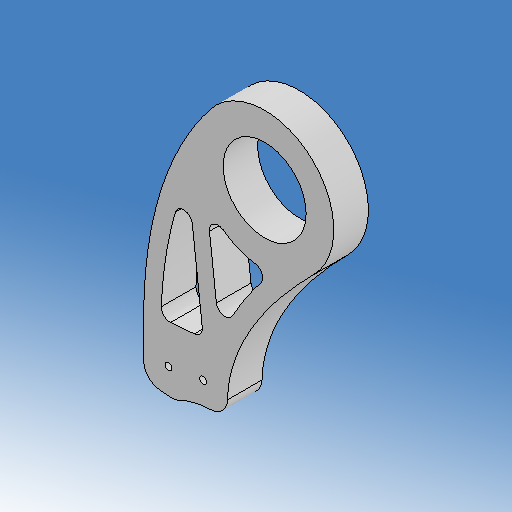
# Autodesk Inventor part: driveshaftsupport_A
Saved by Autodesk Inventor 2025 (Build 290162000, 162)
## iProperties
Created: 2023-03-01
Part Number: driveshaftsupport_A
Material: Generic
Document SubType Name: Modeling
Designer: ralph
Density: 1 g/cm^3
Appearance: Default
Author: ralph
Autodesk Inventor part; units mm, degrees
(part 1 of 2)
ref_plane "YZ Plane" through (0, 0, 0) normal (1, 0, 0) x (0, 1, 0)
ref_plane "XZ Plane" through (0, 0, 0) normal (0, 1, 0) x (-1, 0, 0)
ref_plane "Work Plane1" through (0, 0, 0) normal (0, 0, 1) x (1, 0, 0)
sketch "Sketch1" plane through (0, 0, 0) normal (0, 0, 1) x (1, 0, 0)
  arc A0 (-20.648, -102.4649) -> (-16.3515, -107.2084) centre (-14.4346, -101.1546) ccw
  arc A1 (-10.9828, -109.2489) -> (-16.3515, -107.2084) centre (-31.6865, -155.6385) ccw
  arc A2 (-10.9828, -109.2489) -> (-4.2979, -108.3017) centre (-8.3948, -103.4502) ccw
  arc A3 (0.8876, -104.599) -> (-4.2979, -108.3017) centre (21.0506, -138.319) ccw
  arc A4 (7.2668, -104.5186) -> (0.8876, -104.599) centre (4.1465, -110.049) ccw
  arc A5 (7.2668, -104.5186) -> (24.5776, -101.9869) centre (14.2875, -92.075) ccw
  arc A6 (30.7127, -100.2372) -> (24.5776, -101.9869) centre (29.151, -106.3922) ccw
  arc A7 (43.0033, -105.7359) -> (30.7127, -100.2372) centre (21.0506, -138.319) ccw
  arc A8 (43.0033, -105.7359) -> (57.752, -89.4091) centre (49.2125, -96.52) ccw
  arc A9 (57.752, -7.1109) -> (57.752, -89.4091) centre (107.1678, -48.26) ccw
  arc A10 (57.752, -7.1109) -> (57.752, 7.1109) centre (49.2125, 0) ccw
  arc A11 (57.752, 89.4091) -> (57.752, 7.1109) centre (107.1678, 48.26) ccw
  arc A12 (57.752, 89.4091) -> (46.7209, 107.3496) centre (49.2125, 96.52) ccw
  arc A13 (37.2777, 118.8104) -> (46.7209, 107.3496) centre (44.8601, 115.4372) ccw
  arc A14 (37.2777, 118.8104) -> (27.7131, 132.1679) centre (28.575, 122.682) ccw
  arc A15 (-1.8719, 154.7102) -> (27.7131, 132.1679) centre (25.2222, 159.584) ccw
  arc A16 (-1.8719, 154.7102) -> (-9.0898, 161.7077) centre (-11.1125, 152.4) ccw
  arc A17 (-57.3497, 188.5663) -> (-9.0898, 161.7077) centre (11.1567, 254.8735) ccw
  arc A18 (-57.3497, 188.5663) -> (-61.9125, 190.5) centre (-61.9125, 184.15) ccw
  line L0 (-61.9125, -74.837) -> (-61.9125, 190.5)
  arc A19 (-57.4675, -76.6522) -> (-61.9125, -74.837) centre (-61.9125, -81.187) ccw
  arc A20 (-57.4675, -76.6522) -> (-50.3955, -79.3664) centre (-50.8, -69.85) ccw
  arc A21 (-20.648, -102.4649) -> (-50.3955, -79.3664) centre (-49.1581, -108.4774) ccw
  line L1 (-54.9779, 170.3652) -> (-48.8256, 159.5987)
  arc A22 (-48.8539, 153.2488) -> (-48.8256, 159.5987) centre (-54.339, 156.4482) ccw
  arc A23 (-48.8539, 153.2488) -> (-49.1732, 139.4288) centre (-36.5125, 146.05) ccw
  arc A24 (-49.4382, 133.0844) -> (-49.1732, 139.4288) centre (-54.8001, 136.4861) ccw
  line L2 (-49.4382, 133.0844) -> (-55.0158, 124.2927)
  arc A25 (-57.9437, 125.1431) -> (-55.0158, 124.2927) centre (-56.3562, 125.1431) ccw
  line L3 (-57.9437, 125.1431) -> (-57.9437, 169.5776)
  arc A26 (-54.9779, 170.3652) -> (-57.9437, 169.5776) centre (-56.3562, 169.5776) ccw
  line L4 (-57.9437, 16.3803) -> (-57.9437, 88.2093)
  arc A27 (-48.4371, 93.7191) -> (-57.9437, 88.2093) centre (-51.5937, 88.2093) ccw
  line L5 (-48.4371, 93.7191) -> (25.1122, 51.5817)
  arc A28 (24.9048, 45.9631) -> (25.1122, 51.5817) centre (23.5339, 48.8268) ccw
  line L6 (24.9048, 45.9631) -> (-48.8518, 10.6528)
  arc A29 (-57.9437, 16.3803) -> (-48.8518, 10.6528) centre (-51.5937, 16.3803) ccw
  line L7 (-12.5571, -63.0775) -> (-11.8021, -62.3567)
  arc A30 (-6.8531, -63.0782) -> (-11.8021, -62.3567) centre (-9.6098, -64.6534) ccw
  line L8 (-6.8531, -63.0782) -> (0.9035, -76.6523)
  arc A31 (-1.2505, -78.8251) -> (0.9035, -76.6523) centre (-0.4748, -77.44) ccw
  line L9 (-1.2505, -78.8251) -> (-11.2752, -73.2112)
  arc A32 (-12.5571, -63.0775) -> (-11.2752, -73.2112) centre (-8.1726, -67.6708) ccw
  line L10 (8.063, -43.7132) -> (40.1759, -13.8303)
  arc A33 (42.6746, -15.7078) -> (40.1759, -13.8303) centre (41.2574, -14.9925) ccw
  arc A34 (42.6746, -15.7078) -> (35.0956, -43.2986) centre (107.1678, -48.26) ccw
  arc A35 (28.7606, -49.2125) -> (35.0956, -43.2986) centre (28.7606, -42.8625) ccw
  line L11 (28.7606, -49.2125) -> (10.2259, -49.2125)
  arc A36 (8.063, -43.7132) -> (10.2259, -49.2125) centre (10.2259, -46.0375) ccw
  arc A37 (0.0566, -90.8047) -> (0.0035, -91.7596) centre (14.2875, -92.075) ccw
  arc A38 (-5.1562, -94.1671) -> (0.0035, -91.7596) centre (-3.1707, -91.6895) ccw
  arc A39 (-5.1562, -94.1671) -> (-8.4369, -92.4585) centre (-11.1125, -101.6) ccw
  arc A40 (-12.4439, -88.97) -> (-8.4369, -92.4585) centre (-6.6532, -86.3642) ccw
  line L12 (-12.4439, -88.97) -> (-14.871, -83.5766)
  arc A41 (-12.6476, -81.54) -> (-14.871, -83.5766) centre (-13.4233, -82.9251) ccw
  line L13 (-12.6476, -81.54) -> (-1.5545, -87.7521)
  arc A42 (0.0566, -90.8047) -> (-1.5545, -87.7521) centre (-3.1058, -90.5224) ccw
  line L14 (35.1248, 3.9688) -> (-30.4467, 3.9688)
  arc A43 (-31.8177, 10.0075) -> (-30.4467, 3.9688) centre (-30.4467, 7.1438) ccw
  line L15 (-31.8177, 10.0075) -> (27.4027, 38.3586)
  arc A44 (36.3678, 33.8939) -> (27.4027, 38.3586) centre (30.1446, 32.6312) ccw
  arc A45 (36.3678, 33.8939) -> (42.7868, 15.4863) centre (107.1678, 48.26) ccw
  arc A46 (41.5223, 8.0217) -> (42.7868, 15.4863) centre (37.1279, 12.6056) ccw
  arc A47 (41.5223, 8.0217) -> (40.2476, 6.5665) centre (49.2125, 0) ccw
  arc A48 (35.1248, 3.9688) -> (40.2476, 6.5665) centre (35.1248, 10.3188) ccw
  line L16 (-30.2893, 128.8322) -> (-21.4237, 114.8579)
  arc A49 (-24.1047, 109.982) -> (-21.4237, 114.8579) centre (-24.1047, 113.157) ccw
  line L17 (-24.1047, 109.982) -> (-43.146, 109.982)
  arc A50 (-48.5079, 119.7337) -> (-43.146, 109.982) centre (-43.146, 116.332) ccw
  line L18 (-48.5079, 119.7337) -> (-42.7357, 128.8322)
  arc A51 (-37.1087, 131.7749) -> (-42.7357, 128.8322) centre (-37.3737, 125.4305) ccw
  arc A52 (-37.1087, 131.7749) -> (-35.9163, 131.7749) centre (-36.5125, 146.05) ccw
  arc A53 (-30.2893, 128.8322) -> (-35.9163, 131.7749) centre (-35.6513, 125.4305) ccw
  arc A54 (-26.2357, 155.9757) -> (-36.4489, 160.3374) centre (-36.5125, 146.05) ccw
  arc A55 (-41.934, 163.5368) -> (-36.4489, 160.3374) centre (-36.4206, 166.6873) ccw
  line L19 (-41.934, 163.5368) -> (-43.2662, 165.8683)
  arc A56 (-41.0698, 168.0164) -> (-43.2662, 165.8683) centre (-41.8879, 166.6559) ccw
  arc A57 (-41.0698, 168.0164) -> (-20.6642, 158.6488) centre (11.1567, 254.8735) ccw
  arc A58 (-19.7269, 156.4642) -> (-20.6642, 158.6488) centre (-21.1626, 157.1416) ccw
  arc A59 (-19.7269, 156.4642) -> (-20.2275, 155.1645) centre (-11.1125, 152.4) ccw
  arc A60 (-21.7728, 154.038) -> (-20.2275, 155.1645) centre (-21.7467, 155.6253) ccw
  arc A61 (-26.2357, 155.9757) -> (-21.7728, 154.038) centre (-21.6682, 160.3871) ccw
  arc A62 (39.7212, 90.7404) -> (41.5223, 88.4983) centre (49.2125, 96.52) ccw
  arc A63 (42.7868, 81.0337) -> (41.5223, 88.4983) centre (37.1279, 83.9144) ccw
  arc A64 (42.7868, 81.0337) -> (36.5882, 63.6726) centre (107.1678, 48.26) ccw
  arc A65 (27.2278, 59.5175) -> (36.5882, 63.6726) centre (30.3844, 65.0273) ccw
  line L20 (27.2278, 59.5175) -> (-38.1265, 96.9599)
  arc A66 (-37.2022, 99.9191) -> (-38.1265, 96.9599) centre (-37.3374, 98.3373) ccw
  line L21 (-37.2022, 99.9191) -> (34.8381, 93.7648)
  arc A67 (39.7212, 90.7404) -> (34.8381, 93.7648) centre (34.2976, 87.4378) ccw
  line L22 (-57.9437, -42.8625) -> (-57.9437, -24.653)
  arc A68 (-47.137, -20.1298) -> (-57.9437, -24.653) centre (-51.5937, -24.653) ccw
  line L23 (-47.137, -20.1298) -> (-23.138, -43.7759)
  arc A69 (-25.3663, -49.2125) -> (-23.138, -43.7759) centre (-25.3663, -46.0375) ccw
  line L24 (-25.3663, -49.2125) -> (-51.5937, -49.2125)
  arc A70 (-57.9437, -42.8625) -> (-51.5937, -49.2125) centre (-51.5937, -42.8625) ccw
  arc A71 (33.2333, -92.6915) -> (32.5694, -92.5194) centre (21.0506, -138.319) ccw
  arc A72 (28.0165, -88.1193) -> (32.5694, -92.5194) centre (34.1183, -86.3612) ccw
  arc A73 (28.0165, -88.1193) -> (26.6289, -84.8762) centre (14.2875, -92.075) ccw
  arc A74 (26.6006, -78.5263) -> (26.6289, -84.8762) centre (32.114, -81.6768) ccw
  line L25 (26.6006, -78.5263) -> (34.1483, -65.3178)
  arc A75 (37.0671, -65.7217) -> (34.1483, -65.3178) centre (35.5267, -66.1055) ccw
  arc A76 (37.0671, -65.7217) -> (42.7868, -81.0337) centre (107.1678, -48.26) ccw
  arc A77 (41.5223, -88.4983) -> (42.7868, -81.0337) centre (37.1279, -83.9144) ccw
  arc A78 (41.5223, -88.4983) -> (40.0864, -90.1796) centre (49.2125, -96.52) ccw
  arc A79 (33.2333, -92.6915) -> (40.0864, -90.1796) centre (34.8714, -86.5564) ccw
  line L26 (26.9592, -61.9002) -> (19.8008, -74.4274)
  arc A80 (8.7742, -74.4274) -> (19.8008, -74.4274) centre (14.2875, -71.2769) ccw
  line L27 (8.7742, -74.4274) -> (4.3302, -66.6505)
  arc A81 (9.8436, -57.15) -> (4.3302, -66.6505) centre (9.8436, -63.5) ccw
  line L28 (9.8436, -57.15) -> (24.2025, -57.15)
  arc A82 (26.9592, -61.9002) -> (24.2025, -57.15) centre (24.2025, -60.325) ccw
  line L29 (-36.7375, -3.9687) -> (31.0491, -3.9688)
  arc A83 (33.212, -9.4681) -> (31.0491, -3.9688) centre (31.0491, -7.1437) ccw
  line L30 (33.212, -9.4681) -> (-3.4078, -43.5448)
  arc A84 (-12.1903, -43.4194) -> (-3.4078, -43.5448) centre (-7.7336, -38.8962) ccw
  line L31 (-12.1903, -43.4194) -> (-41.1943, -14.842)
  arc A85 (-36.7375, -3.9687) -> (-41.1943, -14.842) centre (-36.7375, -10.3187) ccw
  arc A86 (-23.8518, 139.4288) -> (-22.4829, 143.3475) centre (-36.5125, 146.05) ccw
  arc A87 (-17.3021, 145.1602) -> (-22.4829, 143.3475) centre (-19.3652, 142.7469) ccw
  arc A88 (-17.3021, 145.1602) -> (-16.4703, 144.5248) centre (-11.1125, 152.4) ccw
  arc A89 (-15.0812, 141.8997) -> (-16.4703, 144.5248) centre (-18.2562, 141.8997) ccw
  line L32 (-15.0812, 141.8997) -> (-15.0812, 125.1431)
  arc A90 (-18.0092, 124.2927) -> (-15.0812, 125.1431) centre (-16.6687, 125.1431) ccw
  line L33 (-18.0092, 124.2927) -> (-23.5868, 133.0844)
  arc A91 (-23.8518, 139.4288) -> (-23.5868, 133.0844) centre (-18.2249, 136.4861) ccw
  circle A92 centre (-11.1125, -101.6) radius 3.175
  circle A93 centre (-11.1125, 152.4) radius 3.175
  circle A94 centre (-50.8, -69.85) radius 3.175
  circle A95 centre (-36.5125, 146.05) radius 7.9375
  circle A96 centre (14.2875, -92.075) radius 7.9375
  circle A97 centre (49.2125, 96.52) radius 3.175
  circle A98 centre (49.2125, 0) radius 3.175
  circle A99 centre (49.2125, -96.52) radius 3.175
  circle A100 centre (3.175, 122.682) radius 3.175
  circle A101 centre (-25.4, -69.85) radius 3.175
  circle A102 centre (28.575, 122.682) radius 3.175
  circle A103 centre (-17.4625, 254) radius 15.9004
  circle A104 centre (6.6997, 178.392) radius 13.97
  arc A105 (-21.0789, 160.5407) -> (-20.5213, 159.7014) centre (6.6997, 178.392) ccw
  arc A106 (-20.5213, 159.7014) -> (-17.7421, 160.6963) centre (-23.3828, 172.0749) ccw
  arc A107 (-17.7421, 160.6963) -> (-16.917, 159.6092) centre (6.6997, 178.392) ccw
  arc A108 (-16.917, 159.6092) -> (-18.6225, 157.1999) centre (-7.4744, 151.1163) ccw
  arc A109 (-18.6225, 157.1999) -> (-17.9641, 156.4371) centre (6.6997, 178.392) ccw
  arc A110 (-17.9641, 156.4371) -> (-15.3315, 157.7724) centre (-22.3539, 168.3543) ccw
  arc A111 (-15.3315, 157.7724) -> (-14.3766, 156.7973) centre (6.6997, 178.392) ccw
  arc A112 (-14.3766, 156.7973) -> (-15.7668, 154.1933) centre (-3.9441, 149.5549) ccw
  arc A113 (-15.7668, 154.1933) -> (-15.018, 153.519) centre (6.6997, 178.392) ccw
  arc A114 (-15.018, 153.519) -> (-12.5735, 155.1738) centre (-20.8667, 164.7921) ccw
  arc A115 (-12.5735, 155.1738) -> (-11.5039, 154.326) centre (6.6997, 178.392) ccw
  arc A116 (-11.5039, 154.326) -> (-12.5567, 151.5683) centre (-0.246, 148.4483) ccw
  arc A117 (-12.5567, 151.5683) -> (-11.7293, 150.9932) centre (6.6997, 178.392) ccw
  arc A118 (-11.7293, 150.9932) -> (-9.5115, 152.9413) centre (-18.9448, 161.4443) ccw
  arc A119 (-9.5115, 152.9413) -> (-8.3441, 152.2343) centre (6.6997, 178.392) ccw
  arc A120 (-8.3441, 152.2343) -> (-9.043, 149.3663) centre (3.5618, 147.8139) ccw
  arc A121 (-9.043, 149.3663) -> (-8.15, 148.8995) centre (6.6997, 178.392) ccw
  arc A122 (-8.15, 148.8995) -> (-6.1939, 151.1101) centre (-16.6185, 158.3639) ccw
  arc A123 (-6.1939, 151.1101) -> (-4.9471, 150.555) centre (6.6997, 178.392) ccw
  arc A124 (-4.9471, 150.555) -> (-5.281, 147.6221) centre (7.4189, 147.6617) ccw
  arc A125 (-5.281, 147.6221) -> (-4.3365, 147.2709) centre (6.6997, 178.392) ccw
  arc A126 (-4.3365, 147.2709) -> (-2.6729, 149.7093) centre (-13.9245, 155.5992) ccw
  arc A127 (-2.6729, 149.7093) -> (-1.3663, 149.3148) centre (6.6997, 178.392) ccw
  arc A128 (-1.3663, 149.3148) -> (-1.33, 146.3632) centre (11.2648, 147.9941) ccw
  arc A129 (-1.33, 146.3632) -> (-0.349, 146.1331) centre (6.6997, 178.392) ccw
  arc A130 (-0.349, 146.1331) -> (0.9959, 148.7607) centre (-10.9052, 153.1941) ccw
  arc A131 (0.9959, 148.7607) -> (2.3416, 148.5331) centre (6.6997, 178.392) ccw
  arc A132 (2.3416, 148.5331) -> (2.7476, 145.6093) centre (15.0387, 148.806) ccw
  arc A133 (2.7476, 145.6093) -> (3.7497, 145.504) centre (6.6997, 178.392) ccw
  arc A134 (3.7497, 145.504) -> (4.7547, 148.2795) centre (-7.6082, 151.1863) ccw
  arc A135 (4.7547, 148.2795) -> (6.1183, 148.2224) centre (6.6997, 178.392) ccw
  arc A136 (6.1183, 148.2224) -> (6.8875, 145.3725) centre (18.681, 150.0844) ccw
  arc A137 (6.8875, 145.3725) -> (7.8949, 145.3936) centre (6.6997, 178.392) ccw
  arc A138 (7.8949, 145.3936) -> (8.5441, 148.2732) centre (-4.0856, 149.6075) ccw
  arc A139 (8.5441, 148.2732) -> (9.9041, 148.3874) centre (6.6997, 178.392) ccw
  arc A140 (9.9041, 148.3874) -> (11.0244, 145.6564) centre (22.1344, 151.8093) ccw
  arc A141 (11.0244, 145.6564) -> (12.0213, 145.8036) centre (6.6997, 178.392) ccw
  arc A142 (12.0213, 145.8036) -> (12.3044, 148.7418) centre (-0.3929, 148.4827) ccw
  arc A143 (12.3044, 148.7418) -> (13.6394, 149.0256) centre (6.6997, 178.392) ccw
  arc A144 (13.6394, 149.0256) -> (15.0932, 146.4565) centre (25.3444, 153.9534) ccw
  arc A145 (15.0932, 146.4565) -> (16.0637, 146.7275) centre (6.6997, 178.392) ccw
  arc A146 (16.0637, 146.7275) -> (15.9764, 149.6781) centre (3.4116, 147.8296) ccw
  arc A147 (15.9764, 149.6781) -> (17.2653, 150.1269) centre (6.6997, 178.392) ccw
  arc A148 (17.2653, 150.1269) -> (19.0296, 147.7603) centre (28.2603, 156.4829) ccw
  arc A149 (19.0296, 147.7603) -> (19.9585, 148.1508) centre (6.6997, 178.392) ccw
  arc A150 (19.9585, 148.1508) -> (19.502, 151.0672) centre (7.268, 147.6585) ccw
  arc A151 (19.502, 151.0672) -> (20.7245, 151.674) centre (6.6997, 178.392) ccw
  arc A152 (20.7245, 151.674) -> (22.7715, 149.5472) centre (30.8363, 159.3579) ccw
  arc A153 (22.7715, 149.5472) -> (23.6442, 150.051) centre (6.6997, 178.392) ccw
  arc A154 (23.6442, 150.051) -> (22.8258, 152.8872) centre (11.1155, 147.9721) ccw
  arc A155 (22.8258, 152.8872) -> (23.9626, 153.6424) centre (6.6997, 178.392) ccw
  arc A156 (23.9626, 153.6424) -> (26.26, 151.789) centre (33.0315, 162.5331) ccw
  arc A157 (26.26, 151.789) -> (27.0626, 152.3982) centre (6.6997, 178.392) ccw
  arc A158 (27.0626, 152.3982) -> (25.8952, 155.1094) centre (14.8933, 148.7654) ccw
  arc A159 (25.8952, 155.1094) -> (26.9284, 156.0012) centre (6.6997, 178.392) ccw
  arc A160 (26.9284, 156.0012) -> (29.44, 154.4503) centre (34.8116, 165.9584) ccw
  arc A161 (29.44, 154.4503) -> (30.1599, 155.1553) centre (6.6997, 178.392) ccw
  arc A162 (30.1599, 155.1553) -> (28.6619, 157.6989) centre (18.5419, 150.0259) ccw
  arc A163 (28.6619, 157.6989) -> (29.5752, 158.7131) centre (6.6997, 178.392) ccw
  arc A164 (29.5752, 158.7131) -> (32.2613, 157.4892) centre (36.1482, 169.5798) ccw
  arc A165 (32.2613, 157.4892) -> (32.8872, 158.2789) centre (6.6997, 178.392) ccw
  arc A166 (32.8872, 158.2789) -> (31.0823, 160.6146) centre (22.0037, 151.7338) ccw
  arc A167 (31.0823, 160.6146) -> (31.8612, 161.7353) centre (6.6997, 178.392) ccw
  arc A168 (31.8612, 161.7353) -> (34.6796, 160.8577) centre (37.0205, 173.3401) ccw
  arc A169 (34.6796, 160.8577) -> (35.2016, 161.7197) centre (6.6997, 178.392) ccw
  arc A170 (35.2016, 161.7197) -> (33.1181, 163.8107) centre (25.2242, 153.8621) ccw
  arc A171 (33.1181, 163.8107) -> (33.7504, 165.0202) centre (6.6997, 178.392) ccw
  arc A172 (33.7504, 165.0202) -> (36.6566, 164.5028) centre (37.4145, 177.1802) ccw
  arc A173 (36.6566, 164.5028) -> (37.0664, 165.4233) centre (6.6997, 178.392) ccw
  arc A174 (37.0664, 165.4233) -> (34.7373, 167.2368) centre (28.1525, 156.3773) ccw
  arc A175 (34.7373, 167.2368) -> (35.2131, 168.516) centre (6.6997, 178.392) ccw
  arc A176 (35.2131, 168.516) -> (38.1611, 168.3669) centre (37.3242, 181.0393) ccw
  arc A177 (38.1611, 168.3669) -> (38.4524, 169.3316) centre (6.6997, 178.392) ccw
  arc A178 (38.4524, 169.3316) -> (35.9143, 170.8388) centre (30.7425, 159.2396) ccw
  arc A179 (35.9143, 170.8388) -> (36.226, 172.1675) centre (6.6997, 178.392) ccw
  arc A180 (36.226, 172.1675) -> (39.1695, 172.3891) centre (36.7509, 184.8567) ccw
  arc A181 (39.1695, 172.3891) -> (39.3376, 173.3827) centre (6.6997, 178.392) ccw
  arc A182 (39.3376, 173.3827) -> (36.6306, 174.5599) centre (32.9533, 162.404) ccw
  arc A183 (36.6306, 174.5599) -> (36.7733, 175.9172) centre (6.6997, 178.392) ccw
  arc A184 (36.7733, 175.9172) -> (39.6658, 176.506) centre (35.7037, 188.5721) ccw
  arc A185 (39.6658, 176.506) -> (39.708, 177.5128) centre (6.6997, 178.392) ccw
  arc A186 (39.708, 177.5128) -> (36.8749, 178.3415) centre (34.7502, 165.8205) ccw
  arc A187 (36.8749, 178.3415) -> (36.8463, 179.706) centre (6.6997, 178.392) ccw
  arc A188 (36.8463, 179.706) -> (39.6423, 180.6526) centre (34.1991, 192.127) ccw
  arc A189 (39.6423, 180.6526) -> (39.558, 181.6567) centre (6.6997, 178.392) ccw
  arc A190 (39.558, 181.6567) -> (36.6433, 182.1238) centre (36.1046, 169.4353) ccw
  arc A191 (36.6433, 182.1238) -> (36.4439, 183.474) centre (6.6997, 178.392) ccw
  arc A192 (36.4439, 183.474) -> (39.0992, 184.7636) centre (32.2608, 195.4653) ccw
  arc A193 (39.0992, 184.7636) -> (38.8897, 185.7492) centre (6.6997, 178.392) ccw
  arc A194 (38.8897, 185.7492) -> (35.9394, 185.8473) centre (36.9953, 173.1913) ccw
  arc A195 (35.9394, 185.8473) -> (35.5724, 187.1618) centre (6.6997, 178.392) ccw
  arc A196 (35.5724, 187.1618) -> (38.0451, 188.7741) centre (29.9194, 198.5343) ccw
  arc A197 (38.0451, 188.7741) -> (37.7137, 189.7257) centre (6.6997, 178.392) ccw
  arc A198 (37.7137, 189.7257) -> (34.7745, 189.4533) centre (37.4082, 177.0293) ccw
  arc A199 (34.7745, 189.4533) -> (34.2456, 190.7114) centre (6.6997, 178.392) ccw
  arc A200 (34.2456, 190.7114) -> (36.4967, 192.6208) centre (27.2118, 201.2857) ccw
  arc A201 (36.4967, 192.6208) -> (36.0487, 193.5234) centre (6.6997, 178.392) ccw
  arc A202 (36.0487, 193.5234) -> (33.1668, 192.8847) centre (37.3369, 180.8889) ccw
  arc A203 (33.1668, 192.8847) -> (32.4844, 194.0667) centre (6.6997, 178.392) ccw
  arc A204 (32.4844, 194.0667) -> (34.4784, 196.2432) centre (24.1807, 203.676) ccw
  arc A205 (34.4784, 196.2432) -> (33.9208, 197.0825) centre (6.6997, 178.392) ccw
  arc A206 (33.9208, 197.0825) -> (31.1416, 196.0876) centre (36.7823, 184.709) ccw
  arc A207 (31.1416, 196.0876) -> (30.3165, 197.1747) centre (6.6997, 178.392) ccw
  arc A208 (30.3165, 197.1747) -> (32.022, 199.584) centre (20.8739, 205.6676) ccw
  arc A209 (32.022, 199.584) -> (31.3636, 200.3468) centre (6.6997, 178.392) ccw
  arc A210 (31.3636, 200.3468) -> (28.731, 199.0115) centre (35.7534, 188.4296) ccw
  arc A211 (28.731, 199.0115) -> (27.7761, 199.9866) centre (6.6997, 178.392) ccw
  arc A212 (27.7761, 199.9866) -> (29.1663, 202.5906) centre (17.3436, 207.229) ccw
  arc A213 (29.1663, 202.5906) -> (28.4175, 203.2649) centre (6.6997, 178.392) ccw
  arc A214 (28.4175, 203.2649) -> (25.973, 201.6101) centre (34.2662, 191.9918) ccw
  arc A215 (25.973, 201.6101) -> (24.9034, 202.4579) centre (6.6997, 178.392) ccw
  arc A216 (24.9034, 202.4579) -> (25.9562, 205.2156) centre (13.6455, 208.3356) ccw
  arc A217 (25.9562, 205.2156) -> (25.1288, 205.7907) centre (6.6997, 178.392) ccw
  arc A218 (25.1288, 205.7907) -> (22.911, 203.8426) centre (32.3443, 195.3396) ccw
  arc A219 (22.911, 203.8426) -> (21.7436, 204.5496) centre (6.6997, 178.392) ccw
  arc A220 (21.7436, 204.5496) -> (22.4425, 207.4176) centre (9.8377, 208.9701) ccw
  arc A221 (22.4425, 207.4176) -> (21.5495, 207.8844) centre (6.6997, 178.392) ccw
  arc A222 (21.5495, 207.8844) -> (19.5934, 205.6738) centre (30.018, 198.4201) ccw
  arc A223 (19.5934, 205.6738) -> (18.3466, 206.2289) centre (6.6997, 178.392) ccw
  arc A224 (18.3466, 206.2289) -> (18.6805, 209.1618) centre (5.9806, 209.1222) ccw
  arc A225 (18.6805, 209.1618) -> (17.736, 209.513) centre (6.6997, 178.392) ccw
  arc A226 (17.736, 209.513) -> (16.0724, 207.0746) centre (27.324, 201.1847) ccw
  arc A227 (16.0724, 207.0746) -> (14.7658, 207.4691) centre (6.6997, 178.392) ccw
  arc A228 (14.7658, 207.4691) -> (14.7295, 210.4207) centre (2.1347, 208.7898) ccw
  arc A229 (14.7295, 210.4207) -> (13.7485, 210.6508) centre (6.6997, 178.392) ccw
  arc A230 (13.7485, 210.6508) -> (12.4036, 208.0232) centre (24.3047, 203.5899) ccw
  arc A231 (12.4036, 208.0232) -> (11.0579, 208.2508) centre (6.6997, 178.392) ccw
  arc A232 (11.0579, 208.2508) -> (10.6519, 211.1746) centre (-1.6392, 207.9779) ccw
  arc A233 (10.6519, 211.1746) -> (9.6498, 211.2799) centre (6.6997, 178.392) ccw
  arc A234 (9.6498, 211.2799) -> (8.6448, 208.5044) centre (21.0077, 205.5976) ccw
  arc A235 (8.6448, 208.5044) -> (7.2812, 208.5616) centre (6.6997, 178.392) ccw
  arc A236 (7.2812, 208.5616) -> (6.512, 211.4114) centre (-5.2815, 206.6995) ccw
  arc A237 (6.512, 211.4114) -> (5.5046, 211.3903) centre (6.6997, 178.392) ccw
  arc A238 (5.5046, 211.3903) -> (4.8554, 208.5107) centre (17.4851, 207.1764) ccw
  arc A239 (4.8554, 208.5107) -> (3.4954, 208.3965) centre (6.6997, 178.392) ccw
  arc A240 (3.4954, 208.3965) -> (2.3751, 211.1275) centre (-8.7349, 204.9746) ccw
  arc A241 (2.3751, 211.1275) -> (1.3782, 210.9803) centre (6.6997, 178.392) ccw
  arc A242 (1.3782, 210.9803) -> (1.0951, 208.0421) centre (13.7924, 208.3012) ccw
  arc A243 (1.0951, 208.0421) -> (-0.2399, 207.7583) centre (6.6997, 178.392) ccw
  arc A244 (-0.2399, 207.7583) -> (-1.6937, 210.3274) centre (-11.9449, 202.8305) ccw
  arc A245 (-1.6937, 210.3274) -> (-2.6642, 210.0564) centre (6.6997, 178.392) ccw
  arc A246 (-2.6642, 210.0564) -> (-2.5769, 207.1058) centre (9.9879, 208.9543) ccw
  arc A247 (-2.5769, 207.1058) -> (-3.8658, 206.657) centre (6.6997, 178.392) ccw
  arc A248 (-3.8658, 206.657) -> (-5.6301, 209.0236) centre (-14.8608, 200.301) ccw
  arc A249 (-5.6301, 209.0236) -> (-6.559, 208.6331) centre (6.6997, 178.392) ccw
  arc A250 (-6.559, 208.6331) -> (-6.1025, 205.7167) centre (6.1315, 209.1254) ccw
  arc A251 (-6.1025, 205.7167) -> (-7.325, 205.1099) centre (6.6997, 178.392) ccw
  arc A252 (-7.325, 205.1099) -> (-9.372, 207.2367) centre (-17.4368, 197.426) ccw
  arc A253 (-9.372, 207.2367) -> (-10.2447, 206.7329) centre (6.6997, 178.392) ccw
  arc A254 (-10.2447, 206.7329) -> (-9.4263, 203.8967) centre (2.284, 208.8118) ccw
  arc A255 (-9.4263, 203.8967) -> (-10.5631, 203.1415) centre (6.6997, 178.392) ccw
  arc A256 (-10.5631, 203.1415) -> (-12.8605, 204.9949) centre (-19.632, 194.2508) ccw
  arc A257 (-12.8605, 204.9949) -> (-13.6631, 204.3857) centre (6.6997, 178.392) ccw
  arc A258 (-13.6631, 204.3857) -> (-12.4957, 201.6745) centre (-1.4938, 208.0185) ccw
  arc A259 (-12.4957, 201.6745) -> (-13.5289, 200.7827) centre (6.6997, 178.392) ccw
  arc A260 (-13.5289, 200.7827) -> (-16.0405, 202.3336) centre (-21.4121, 190.8255) ccw
  arc A261 (-16.0405, 202.3336) -> (-16.7604, 201.6286) centre (6.6997, 178.392) ccw
  arc A262 (-16.7604, 201.6286) -> (-15.2624, 199.0851) centre (-5.1424, 206.758) ccw
  arc A263 (-15.2624, 199.0851) -> (-16.1757, 198.0708) centre (6.6997, 178.392) ccw
  arc A264 (-16.1757, 198.0708) -> (-18.8618, 199.2947) centre (-22.7487, 187.2041) ccw
  arc A265 (-18.8618, 199.2947) -> (-19.4877, 198.505) centre (6.6997, 178.392) ccw
  arc A266 (-19.4877, 198.505) -> (-17.6828, 196.1693) centre (-8.6042, 205.0501) ccw
  arc A267 (-17.6828, 196.1693) -> (-18.4617, 195.0486) centre (6.6997, 178.392) ccw
  arc A268 (-18.4617, 195.0486) -> (-21.2801, 195.9262) centre (-23.621, 183.4438) ccw
  arc A269 (-21.2801, 195.9262) -> (-21.8021, 195.0643) centre (6.6997, 178.392) ccw
  arc A270 (-21.8021, 195.0643) -> (-19.7186, 192.9732) centre (-11.8247, 202.9218) ccw
  arc A271 (-19.7186, 192.9732) -> (-20.3509, 191.7637) centre (6.6997, 178.392) ccw
  arc A272 (-20.3509, 191.7637) -> (-23.2571, 192.2811) centre (-24.015, 179.6037) ccw
  arc A273 (-23.2571, 192.2811) -> (-23.6669, 191.3606) centre (6.6997, 178.392) ccw
  arc A274 (-23.6669, 191.3606) -> (-21.3378, 189.5471) centre (-14.753, 200.4066) ccw
  arc A275 (-21.3378, 189.5471) -> (-21.8136, 188.2679) centre (6.6997, 178.392) ccw
  arc A276 (-21.8136, 188.2679) -> (-24.7616, 188.417) centre (-23.9247, 175.7446) ccw
  arc A277 (-24.7616, 188.417) -> (-25.0529, 187.4523) centre (6.6997, 178.392) ccw
  arc A278 (-25.0529, 187.4523) -> (-22.5149, 185.9451) centre (-17.343, 197.5443) ccw
  arc A279 (-22.5149, 185.9451) -> (-22.8265, 184.6164) centre (6.6997, 178.392) ccw
  arc A280 (-22.8265, 184.6164) -> (-25.77, 184.3948) centre (-23.3514, 171.9272) ccw
  arc A281 (-25.77, 184.3948) -> (-25.9381, 183.4012) centre (6.6997, 178.392) ccw
  arc A282 (-25.9381, 183.4012) -> (-23.2311, 182.224) centre (-19.5538, 194.3799) ccw
  arc A283 (-23.2311, 182.224) -> (-23.3738, 180.8667) centre (6.6997, 178.392) ccw
  arc A284 (-23.3738, 180.8667) -> (-26.2663, 180.2779) centre (-22.3042, 168.2118) ccw
  arc A285 (-26.2663, 180.2779) -> (-26.3085, 179.2711) centre (6.6997, 178.392) ccw
  arc A286 (-26.3085, 179.2711) -> (-23.4754, 178.4424) centre (-21.3507, 190.9634) ccw
  arc A287 (-23.4754, 178.4424) -> (-23.4468, 177.0779) centre (6.6997, 178.392) ccw
  arc A288 (-23.4468, 177.0779) -> (-26.2428, 176.1313) centre (-20.7996, 164.6569) ccw
  arc A289 (-26.2428, 176.1313) -> (-26.1585, 175.1272) centre (6.6997, 178.392) ccw
  arc A290 (-26.1585, 175.1272) -> (-23.2438, 174.6601) centre (-22.7051, 187.3486) ccw
  arc A291 (-23.2438, 174.6601) -> (-23.0444, 173.3099) centre (6.6997, 178.392) ccw
  arc A292 (-23.0444, 173.3099) -> (-25.6997, 172.0203) centre (-18.8613, 161.3186) ccw
  arc A293 (-25.6997, 172.0203) -> (-25.4902, 171.0347) centre (6.6997, 178.392) ccw
  arc A294 (-25.4902, 171.0347) -> (-22.5399, 170.9366) centre (-23.5958, 183.5926) ccw
  arc A295 (-22.5399, 170.9366) -> (-22.1729, 169.6221) centre (6.6997, 178.392) ccw
  arc A296 (-22.1729, 169.6221) -> (-24.6456, 168.0098) centre (-16.5199, 158.2496) ccw
  arc A297 (-24.6456, 168.0098) -> (-24.3142, 167.0582) centre (6.6997, 178.392) ccw
  arc A298 (-24.3142, 167.0582) -> (-21.375, 167.3307) centre (-24.0087, 179.7546) ccw
  arc A299 (-21.375, 167.3307) -> (-20.8461, 166.0725) centre (6.6997, 178.392) ccw
  arc A300 (-20.8461, 166.0725) -> (-23.0972, 164.1631) centre (-13.8123, 155.4982) ccw
  arc A301 (-23.0972, 164.1631) -> (-22.6492, 163.2605) centre (6.6997, 178.392) ccw
  arc A302 (-22.6492, 163.2605) -> (-19.7673, 163.8992) centre (-23.9374, 175.895) ccw
  arc A303 (-19.7673, 163.8992) -> (-19.0849, 162.7172) centre (6.6997, 178.392) ccw
  arc A304 (-19.0849, 162.7172) -> (-21.0789, 160.5407) centre (-10.7812, 153.1079) ccw
  arc A305 (57.752, 89.4091) -> (57.752, 7.1109) centre (107.1678, 48.26) ccw
  arc A306 (57.752, 89.4091) -> (46.7209, 107.3496) centre (49.2125, 96.52) ccw
  arc A307 (37.2777, 118.8104) -> (46.7209, 107.3496) centre (44.8601, 115.4372) ccw
  arc A308 (37.2777, 118.8104) -> (26.151, 131.8934) centre (28.575, 122.682) ccw
  arc A309 (-24.0778, 153.0864) -> (26.151, 131.8934) centre (14.7867, 175.0785) ccw
  line L34 (-61.9125, -190.5) -> (-61.9125, 190.5)
  arc A310 (47.014, -107.4129) -> (-13.8897, -132.1844) centre (35.2441, -165.7303) ccw
  arc A311 (47.014, -107.4129) -> (57.752, -89.4091) centre (49.2125, -96.52) ccw
  arc A312 (57.752, -7.1109) -> (57.752, -89.4091) centre (107.1678, -48.26) ccw
  arc A313 (57.752, -7.1109) -> (57.752, 7.1109) centre (49.2125, 0) ccw
  arc A314 (42.6746, -15.7078) -> (35.0956, -43.2986) centre (107.1678, -48.26) ccw
  arc A315 (28.7606, -49.2125) -> (35.0956, -43.2986) centre (28.7606, -42.8625) ccw
  line L35 (28.7606, -49.2125) -> (6.1896, -49.2125)
  arc A316 (5.1081, -46.4628) -> (6.1896, -49.2125) centre (6.1896, -47.625) ccw
  line L36 (5.1081, -46.4628) -> (40.1759, -13.8303)
  arc A317 (42.6746, -15.7078) -> (40.1759, -13.8303) centre (41.2574, -14.9925) ccw
  line L37 (33.212, -9.4681) -> (-3.4078, -43.5448)
  arc A318 (-12.1903, -43.4194) -> (-3.4078, -43.5448) centre (-7.7336, -38.8962) ccw
  line L38 (-12.1903, -43.4194) -> (-46.712, -9.4054)
  arc A319 (-44.4837, -3.9687) -> (-46.712, -9.4054) centre (-44.4837, -7.1437) ccw
  line L39 (-44.4837, -3.9687) -> (31.0491, -3.9688)
  arc A320 (33.212, -9.4681) -> (31.0491, -3.9688) centre (31.0491, -7.1437) ccw
  line L40 (35.1248, 3.9688) -> (-37.4391, 3.9688)
  arc A321 (-38.1246, 6.9881) -> (-37.4391, 3.9688) centre (-37.4391, 5.5563) ccw
  line L41 (-38.1246, 6.9881) -> (27.4027, 38.3586)
  arc A322 (36.3678, 33.8939) -> (27.4027, 38.3586) centre (30.1446, 32.6312) ccw
  arc A323 (36.3678, 33.8939) -> (42.7868, 15.4863) centre (107.1678, 48.26) ccw
  arc A324 (41.5223, 8.0217) -> (42.7868, 15.4863) centre (37.1279, 12.6056) ccw
  arc A325 (41.5223, 8.0217) -> (40.2476, 6.5665) centre (49.2125, 0) ccw
  arc A326 (35.1248, 3.9688) -> (40.2476, 6.5665) centre (35.1248, 10.3188) ccw
  line L42 (24.9048, 45.9631) -> (-48.8518, 10.6528)
  arc A327 (-57.9437, 16.3803) -> (-48.8518, 10.6528) centre (-51.5937, 16.3803) ccw
  line L43 (-57.9437, 16.3803) -> (-57.9437, 93.6874)
  arc A328 (-53.1904, 96.4423) -> (-57.9437, 93.6874) centre (-54.7687, 93.6874) ccw
  line L44 (-53.1904, 96.4423) -> (25.1122, 51.5817)
  arc A329 (24.9048, 45.9631) -> (25.1122, 51.5817) centre (23.5339, 48.8268) ccw
  line L45 (27.2278, 59.5175) -> (-38.1265, 96.9599)
  arc A330 (-37.2022, 99.9191) -> (-38.1265, 96.9599) centre (-37.3374, 98.3373) ccw
  line L46 (-37.2022, 99.9191) -> (34.8381, 93.7648)
  arc A331 (39.7212, 90.7404) -> (34.8381, 93.7648) centre (34.2976, 87.4378) ccw
  arc A332 (39.7212, 90.7404) -> (41.5223, 88.4983) centre (49.2125, 96.52) ccw
  arc A333 (42.7868, 81.0337) -> (41.5223, 88.4983) centre (37.1279, 83.9144) ccw
  arc A334 (42.7868, 81.0337) -> (36.5882, 63.6726) centre (107.1678, 48.26) ccw
  arc A335 (27.2278, 59.5175) -> (36.5882, 63.6726) centre (30.3844, 65.0273) ccw
  line L47 (-24.1047, 109.982) -> (-48.9203, 109.982)
  arc A336 (-51.6013, 114.8579) -> (-48.9203, 109.982) centre (-48.9203, 113.157) ccw
  line L48 (-51.6013, 114.8579) -> (-42.7357, 128.8322)
  arc A337 (-37.1087, 131.7749) -> (-42.7357, 128.8322) centre (-37.3737, 125.4305) ccw
  arc A338 (-37.1087, 131.7749) -> (-35.9163, 131.7749) centre (-36.5125, 146.05) ccw
  arc A339 (-30.2893, 128.8322) -> (-35.9163, 131.7749) centre (-35.6513, 125.4305) ccw
  line L49 (-30.2893, 128.8322) -> (-21.4237, 114.8579)
  arc A340 (-24.1047, 109.982) -> (-21.4237, 114.8579) centre (-24.1047, 113.157) ccw
  line L50 (-49.4382, 133.0844) -> (-55.0158, 124.2927)
  arc A341 (-57.9437, 125.1431) -> (-55.0158, 124.2927) centre (-56.3562, 125.1431) ccw
  line L51 (-57.9437, 125.1431) -> (-57.9437, 162.8921)
  arc A342 (-55.1499, 163.9241) -> (-57.9437, 162.8921) centre (-56.3562, 162.8921) ccw
  arc A343 (-55.1499, 163.9241) -> (-51.0336, 159.8453) centre (-28.3854, 186.8185) ccw
  arc A344 (-49.3924, 152.2338) -> (-51.0336, 159.8453) centre (-55.1168, 154.9822) ccw
  arc A345 (-49.3924, 152.2338) -> (-49.1732, 139.4288) centre (-36.5125, 146.05) ccw
  arc A346 (-49.4382, 133.0844) -> (-49.1732, 139.4288) centre (-54.8001, 136.4861) ccw
  circle A347 centre (-36.5125, 146.05) radius 7.9375
  circle A348 centre (28.575, 122.682) radius 3.175
  circle A349 centre (3.175, 122.682) radius 3.175
  circle A350 centre (49.2125, 0) radius 3.175
  circle A351 centre (49.2125, 96.52) radius 3.175
  line L52 (-12.9337, 116.2924) -> (-25.1948, 135.619)
  arc A352 (-25.1202, 137.4275) -> (-25.1948, 135.619) centre (-23.8544, 136.4694) ccw
  arc A353 (-25.1202, 137.4275) -> (-24.8809, 137.7531) centre (-36.5125, 146.05) ccw
  arc A354 (-22.4641, 137.9519) -> (-24.8809, 137.7531) centre (-23.5885, 136.8312) ccw
  arc A355 (-22.4641, 137.9519) -> (-9.737, 128.5533) centre (14.7867, 175.0785) ccw
  arc A356 (-6.3488, 122.8343) -> (-9.737, 128.5533) centre (-12.698, 122.9359) ccw
  arc A357 (-6.3488, 122.8343) -> (-6.2364, 121.2154) centre (3.175, 122.682) ccw
  arc A358 (-7.6894, 116.1052) -> (-6.2364, 121.2154) centre (-12.5107, 120.2377) ccw
  line L53 (-7.6894, 116.1052) -> (-7.8421, 115.927)
  arc A359 (-12.9337, 116.2924) -> (-7.8421, 115.927) centre (-10.2528, 117.9933) ccw
  circle A360 centre (-50.8, -69.85) radius 3.175
  circle A361 centre (49.2125, -96.52) radius 3.175
  circle A362 centre (-24.3783, -125.0234) radius 6.35
  circle A363 centre (14.2875, -92.075) radius 7.9375
  circle A364 centre (-25.4, -69.85) radius 3.175
  line L54 (-57.9437, -42.8625) -> (-57.9437, -17.0675)
  arc A365 (-52.5404, -14.8058) -> (-57.9437, -17.0675) centre (-54.7687, -17.0675) ccw
  line L55 (-52.5404, -14.8058) -> (-23.138, -43.7759)
  arc A366 (-25.3663, -49.2125) -> (-23.138, -43.7759) centre (-25.3663, -46.0375) ccw
  line L56 (-25.3663, -49.2125) -> (-51.5937, -49.2125)
  arc A367 (-57.9437, -42.8625) -> (-51.5937, -49.2125) centre (-51.5937, -42.8625) ccw
  line L57 (35.7386, -90.8044) -> (32.5182, -90.3945)
  arc A368 (27.4638, -86.5506) -> (32.5182, -90.3945) centre (33.3199, -84.0953) ccw
  arc A369 (27.4638, -86.5506) -> (26.6289, -84.8762) centre (14.2875, -92.075) ccw
  arc A370 (26.6006, -78.5263) -> (26.6289, -84.8762) centre (32.114, -81.6768) ccw
  line L58 (26.6006, -78.5263) -> (32.2564, -68.6287)
  arc A371 (38.0507, -69.2801) -> (32.2564, -68.6287) centre (35.0131, -70.204) ccw
  arc A372 (38.0507, -69.2801) -> (42.7868, -81.0337) centre (107.1678, -48.26) ccw
  arc A373 (41.5223, -88.4983) -> (42.7868, -81.0337) centre (37.1279, -83.9144) ccw
  arc A374 (41.5223, -88.4983) -> (41.1484, -88.8742) centre (49.2125, -96.52) ccw
  arc A375 (35.7386, -90.8044) -> (41.1484, -88.8742) centre (36.5404, -84.5052) ccw
  arc A376 (-28.7026, -113.0823) -> (-28.7198, -113.0886) centre (-24.3783, -125.0234) ccw
  arc A377 (-34.7309, -112.1782) -> (-28.7198, -113.0886) centre (-30.8906, -107.1211) ccw
  line L59 (-34.7309, -112.1782) -> (-48.9893, -101.3504)
  arc A378 (-49.1247, -91.3419) -> (-48.9893, -101.3504) centre (-45.149, -96.2933) ccw
  line L60 (-49.1247, -91.3419) -> (-34.7812, -79.8249)
  arc A379 (-28.6433, -78.8058) -> (-34.7812, -79.8249) centre (-30.8055, -84.7764) ccw
  arc A380 (-28.6433, -78.8058) -> (-22.7544, -79.0002) centre (-25.4, -69.85) ccw
  arc A381 (-18.7775, -82.7585) -> (-22.7544, -79.0002) centre (-21.8725, -82.0503) ccw
  line L61 (-18.7775, -82.7585) -> (-24.6748, -108.5283)
  arc A382 (-28.7026, -113.0823) -> (-24.6748, -108.5283) centre (-30.8648, -107.1118) ccw
  arc A383 (-2.0508, -103.9163) -> (-14.7048, -113.6056) centre (35.2441, -165.7303) ccw
  arc A384 (-17.3507, -112.1053) -> (-14.7048, -113.6056) centre (-15.8032, -112.4594) ccw
  line L62 (-17.3507, -112.1053) -> (-7.245, -67.9461)
  arc A385 (-4.3192, -67.5126) -> (-7.245, -67.9461) centre (-5.6975, -68.3002) ccw
  line L63 (-4.3192, -67.5126) -> (1.9744, -78.5263)
  arc A386 (1.9461, -84.8762) -> (1.9744, -78.5263) centre (-3.539, -81.6768) ccw
  arc A387 (1.9461, -84.8762) -> (0.7054, -96.5087) centre (14.2875, -92.075) ccw
  arc A388 (-2.0508, -103.9163) -> (0.7054, -96.5087) centre (-5.3312, -98.4793) ccw
  arc A389 (-37.0406, -124.0456) -> (-35.2791, -131.5397) centre (-24.3783, -125.0234) ccw
  arc A390 (-36.5242, -139.5557) -> (-35.2791, -131.5397) centre (-40.7295, -134.7978) ccw
  arc A391 (-36.5242, -139.5557) -> (-52.1016, -157.6717) centre (21.5017, -205.2058) ccw
  arc A392 (-57.9438, -155.9492) -> (-52.1016, -157.6717) centre (-54.7688, -155.9492) ccw
  line L64 (-57.9438, -155.9492) -> (-57.9438, -110.9151)
  arc A393 (-52.8486, -108.3865) -> (-57.9438, -110.9151) centre (-54.7688, -110.9151) ccw
  line L65 (-52.8486, -108.3865) -> (-39.5314, -118.4996)
  arc A394 (-37.0406, -124.0456) -> (-39.5314, -118.4996) centre (-43.3717, -123.5567) ccw
  line L66 (26.9592, -61.9002) -> (19.8008, -74.4274)
  arc A395 (8.7742, -74.4274) -> (19.8008, -74.4274) centre (14.2875, -71.2769) ccw
  line L67 (8.7742, -74.4274) -> (1.6158, -61.9002)
  arc A396 (4.3725, -57.15) -> (1.6158, -61.9002) centre (4.3725, -60.325) ccw
  line L68 (4.3725, -57.15) -> (24.2025, -57.15)
  arc A397 (26.9592, -61.9002) -> (24.2025, -57.15) centre (24.2025, -60.325) ccw
  circle A398 centre (-17.4625, 254) radius 25.4
  spline S0 degree 3 poles (-29.446, 168.6111) (-36.8238, 190.9821) (-18.8707, 216.6708) (0.498, 236.0395) knots 0 0 0 0 1 1 1 1
  line L69 (-17.4625, 254) -> (0.498, 236.0395) construction
  line L70 (-17.4625, 254) -> (7.9375, 254) construction
  line L71 (-61.9125, 190.5) -> (-61.9125, 238.0996) construction
  line L72 (-61.9125, 238.0996) -> (-37.5415, 269.5562) construction
  spline S1 degree 2 poles (-61.9125, 190.5) (-61.9125, 238.0996) (-37.5415, 269.5562) knots 1 1 1 2 2 2
  line L73 (-17.4625, 254) -> (9.2096, 254) construction
  line L74 (-61.9125, 190.5) -> (-61.9125, 171.704)
  line L75 (-61.9125, 171.704) -> (-29.446, 168.6111)
  line L76 (-61.9125, 190.5) -> (-61.9125, 171.704)
  line L77 (-61.9125, 181.102) -> (-31.1206, 178.1687)
  circle A399 centre (-52.7964, 180.2336) radius 3.175
  circle A400 centre (-40.0964, 179.0237) radius 3.175
  spline S2 degree 4 poles (-24.0778, 153.0864) (-27.2352, 158.6662) (-34.1556, 163.6823) (-33.0429, 169.7473) (-31.5921, 176.0063) knots 0 0 0 0 0 0.80197 0.80197 0.80197 0.80197 0.80197
  spline S3 degree 4 poles (-31.5921, 176.0063) (-31.2339, 177.5519) (-30.855, 179.1092) (-30.5714, 180.6655) (-30.5714, 182.1987) knots 0 0 0 0 0 1 1 1 1 1
  arc A401 (-30.5714, 182.1987) -> (-40.0964, 191.7237) centre (-40.0964, 182.1987) ccw
  line L78 (-40.0964, 191.7237) -> (-61.9125, 190.5)
  line L79 (-61.9125, -190.5) -> (-40.0964, -191.7237)
  arc A402 (-40.0964, -191.7237) -> (-30.5714, -182.1987) centre (-40.0964, -182.1987) ccw
  spline S4 degree 4 poles (-30.5714, -182.1987) (-30.5714, -172.2165) (-43.0585, -166.7432) (-23.0557, -145.6096) (-13.8897, -132.1844) knots -1 -1 -1 -1 -1 0 0 0 0 0
  circle A403 centre (-40.0964, -182.1987) radius 2.413
  circle A404 centre (-52.7964, -180.2336) radius 2.413
  ellipse E0 centre (-17.2358, 253.9919) end of major axis (-28.8322, 259.1701) minor radius 12.7
  point P0 (0, 0)
  point P1 (-25.8221, 200.765)
  point P2 (-61.9125, 181.102)
  dimension "d0" = 50.8
  dimension "d1" = 45
  dimension "d3" = 18.796
  dimension "d4" = 6.35
  dimension "d5" = 6.35
  dimension "d6" = 12.7
  dimension "d7" = 9.1161
  constraints: 14 end point, 3 centre point, 3 point on circle, 3 point on line, 2 collinear, 2 horizontal, 2 midpoint, 1 coincident, 1 equal length, 1 parallel, 1 tangent, 9 other
  measures "d0" diameter of A398
  measures "d1" angle of L69 L70
  measures "d3" distance of L0.end L74.end
  measures "d4" diameter of A399
  measures "d5" diameter of A400
  measures "d6" horizontal distance of A400.centre A399.centre
  measures "d7" horizontal distance of point (-61.912, 181.102) A399.centre
extrude "Extrusion1" add sketch "Sketch1" along normal blind 12.7 contours L0 L77 A399 A17 S2 L75 | L0 A18 A17 A399 L77 | S2 A17 L75 | L78 A401 S0 L77 A400 A17 A399 A18 | S1 A398 S0 A401 L78 | A17 S2 S3 S0 | A17 L77 A400 S0 S3 S2 | A398 | A399 A17 L77 picked at (-48.5049, 180.0172)